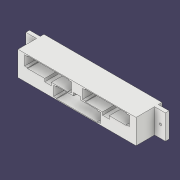
# Autodesk Inventor part: BP011
Saved by Autodesk Inventor 2017 SP1 (Build 210196100, 196)
## iProperties
Created: 2018-06-18
Part Number: BP011
Material: ABS Plastic
Document SubType Name: Modeling
Designer: Zach
Density: 1.06 g/cm^3
Appearance: CR White
Author: Zach
Autodesk Inventor part; units mm, degrees
ref_plane "YZ Plane" through (0, 0, 0) normal (1, 0, 0) x (0, 1, 0)
ref_plane "XZ Plane" through (0, 0, 0) normal (0, 1, 0) x (-1, 0, 0)
ref_plane "XY Plane" through (0, 0, 0) normal (0, 0, 1) x (1, 0, 0)
sketch "Sketch1" plane through (0, 0, 0) normal (0, 0, 1) x (1, 0, 0)
  line L0 (0, 0) -> (190, 0)
  line L1 (190, 0) -> (190, 35)
  line L2 (190, 35) -> (0, 35)
  line L3 (0, 35) -> (0, 0)
  circle A0 centre (7.5, 17.5) radius 1.5
  circle A1 centre (182.5, 17.5) radius 1.5
  point P0 (0, 17.5)
  dimension "d0" = 190
  dimension "d1" = 35
  dimension "d2" = 3
  dimension "d3" = 7.5
  dimension "d4" = 3
  dimension "d5" = 7.5
  constraints: 8 end point, 2 centre point, 2 horizontal alignment, 2 parallel, 1 horizontal, 1 midpoint, 1 perpendicular
  measures "d0" distance of L2.end L1.end
  measures "d1" distance of L1.end L0.end
  measures "d2" diameter of A0
  measures "d3" distance from line of L3 A0.centre
  measures "d4" diameter of A1
  measures "d5" distance from line of L1 A1.centre
extrude "Extrusion1" add sketch "Sketch1" along normal blind 5
sketch "Sketch2" plane through (0, 0, 0) normal (0, 0, -1) x (-1, 0, 0)
  line L0 (0, 0) -> (-190, 0) projected
  line L1 (-190, 35) -> (0, 35) projected
  line L2 (-15.5, 0) -> (-174.5, 0)
  line L3 (-174.5, 0) -> (-174.5, 35)
  line L4 (-174.5, 35) -> (-15.5, 35)
  line L5 (-15.5, 35) -> (-15.5, 0)
  point P0 (-95, 0)
  dimension "d8" = 159
  constraints: 8 end point, 2 midpoint, 2 parallel, 2 point on line, 1 horizontal, 1 perpendicular
  measures "d8" distance between parallel lines of L5 L3
extrude "Extrusion2" add sketch "Sketch2" along normal blind 5
sketch "Sketch3" plane through (0, 0, 5) normal (0, 0, 1) x (1, 0, 0)
  circle A0 centre (182.5, 17.5) radius 1.5 projected
  circle A1 centre (7.5, 17.5) radius 1.5 projected
  line L0 (0, 0) -> (190, 0) projected
  line L1 (190, 0) -> (190, 35) projected
  line L2 (190, 35) -> (0, 35) projected
  line L3 (0, 35) -> (0, 0) projected
  line L4 (1, 34) -> (189, 34)
  line L5 (189, 34) -> (189, 1)
  line L6 (189, 1) -> (1, 1)
  line L7 (1, 1) -> (1, 34)
  dimension "d11" = 1
  constraints: 8 end point, 3 other
  measures "d11" distance between parallel lines of L2 L4
extrude "Extrusion3" cut sketch "Sketch3" against normal through all contours L3 L2 L1 L0
sketch "Sketch4" plane through (0, 0, 5) normal (0, 0, 1) x (1, 0, 0)
  line L0 (41, 27) -> (71, 27)
  line L1 (71, 27) -> (71, 8)
  line L2 (71, 8) -> (41, 8)
  line L3 (41, 8) -> (41, 27)
  line L4 (86, 27) -> (116, 27)
  line L5 (116, 27) -> (116, 8)
  line L6 (116, 8) -> (86, 8)
  line L7 (86, 8) -> (86, 27)
  line L8 (131, 27) -> (149, 27)
  line L9 (149, 27) -> (149, 8)
  line L10 (149, 8) -> (131, 8)
  line L11 (131, 8) -> (131, 27)
  line L12 (41, 17.5) -> (149, 17.5) construction
  line L13 (189, 34) -> (1, 34) projected
  circle A0 centre (7.5, 17.5) radius 1.5 projected
  point P0 (0, 0)
  point P1 (95, 17.5)
  point P2 (95, 34)
  dimension "d14" = 30
  dimension "d15" = 19
  dimension "d16" = 30
  dimension "d17" = 19
  dimension "d18" = 18
  dimension "d19" = 19
  dimension "d20" = 15
  dimension "d21" = 15
  constraints: 26 end point, 6 parallel, 4 midpoint, 3 horizontal, 3 perpendicular, 2 point on line, 1 horizontal alignment, 1 vertical alignment
  measures "d14" distance of L1.end L2.end
  measures "d15" distance of L0.end L1.end
  measures "d16" distance of L5.end L6.end
  measures "d17" distance of L4.end L5.end
  measures "d18" distance of L9.end L10.end
  measures "d19" distance of L8.end L9.end
  measures "d20" distance between parallel lines of L1 L7
  measures "d21" distance between parallel lines of L11 L5
extrude "Extrusion4" cut sketch "Sketch4" against normal through all contours L0 L1 L2 L3 | L4 L5 L6 L7 | L8 L9 L10 L11
sketch "Sketch5" plane through (0, 0, 5) normal (0, 0, 1) x (1, 0, 0)
  line L0 (41, 27) -> (41, 8) projected
  line L1 (41, 8) -> (71, 8) projected
  line L2 (71, 8) -> (71, 27) projected
  line L3 (71, 27) -> (41, 27) projected
  line L4 (131, 27) -> (131, 8) projected
  line L5 (131, 8) -> (149, 8) projected
  line L6 (149, 8) -> (149, 27) projected
  line L7 (149, 27) -> (131, 27) projected
  line L8 (86, 27) -> (86, 8) projected
  line L9 (86, 8) -> (116, 8) projected
  line L10 (116, 8) -> (116, 27) projected
  line L11 (116, 27) -> (86, 27) projected
  line L12 (174.5, 1) -> (15.5, 1) projected
  line L13 (15.5, 1) -> (15.5, 34) projected
  line L14 (15.5, 34) -> (174.5, 34) projected
  line L15 (174.5, 34) -> (174.5, 1) projected
  point P0 (0, 0)
extrude "Extrusion5" add sketch "Sketch5" along normal blind 25
sketch "Sketch6" plane through (0, 0, -5) normal (0, 0, -1) x (-1, 0, 0)
  line L0 (-71, 27) -> (-41, 27) projected
  line L1 (-41, 27) -> (-41, 8) projected
  line L2 (-71, 8) -> (-71, 27) projected
  line L3 (-86, 27) -> (-86, 8) projected
  line L4 (-116, 27) -> (-86, 27) projected
  line L5 (-116, 8) -> (-116, 27) projected
  line L6 (-41, 25) -> (-36, 25)
  line L7 (-36, 25) -> (-36, 10)
  line L8 (-36, 10) -> (-41, 10)
  line L9 (-41, 10) -> (-41, 25)
  line L10 (-71, 25) -> (-76, 25)
  line L11 (-76, 25) -> (-76, 10)
  line L12 (-76, 10) -> (-71, 10)
  line L13 (-71, 10) -> (-71, 25)
  line L14 (-86, 25) -> (-81, 25)
  line L15 (-81, 25) -> (-81, 10)
  line L16 (-81, 10) -> (-86, 10)
  line L17 (-86, 10) -> (-86, 25)
  line L18 (-116, 25) -> (-121, 25)
  line L19 (-121, 25) -> (-121, 10)
  line L20 (-121, 10) -> (-116, 10)
  line L21 (-116, 10) -> (-116, 25)
  point P0 (0, 0)
  point P1 (-41, 17.5)
  dimension "d26" = 15
  dimension "d27" = 5
  dimension "d28" = 5
  dimension "d29" = 5
  dimension "d30" = 5
  constraints: 32 end point, 8 parallel, 6 horizontal alignment, 4 horizontal, 4 perpendicular, 4 point on line, 2 midpoint
  measures "d26" distance of L6.end L7.end
  measures "d27" distance of L6.start L6.end
  measures "d28" distance of L10.start L10.end
  measures "d29" distance of L14.start L14.end
  measures "d30" distance of L18.start L18.end
extrude "Extrusion6" cut sketch "Sketch6" against normal blind 22
sketch "Sketch10" plane through (0, 0, 30) normal (0, 0, 1) x (1, 0, 0)
  line L0 (86, 27) -> (116, 27) projected
  line L1 (116, 27) -> (116, 8) projected
  line L2 (116, 8) -> (86, 8) projected
  line L3 (86, 8) -> (86, 27) projected
  line L4 (41, 27) -> (71, 27) projected
  line L5 (71, 27) -> (71, 8) projected
  line L6 (71, 8) -> (41, 8) projected
  line L7 (41, 8) -> (41, 27) projected
  line L8 (131, 27) -> (149, 27) projected
  line L9 (149, 27) -> (149, 8) projected
  line L10 (149, 8) -> (131, 8) projected
  line L11 (131, 8) -> (131, 27) projected
  line L12 (15.5, 1) -> (174.5, 1) projected
  line L13 (174.5, 1) -> (174.5, 34) projected
  line L14 (174.5, 34) -> (15.5, 34) projected
  line L15 (15.5, 34) -> (15.5, 1) projected
  point P0 (0, 0)
extrude "Extrusion7" add sketch "Sketch10" against normal blind 35 contours L0 L1 L2 L3 | L4 L5 L6 L7 | L8 L9 L10 L11 | L15 L14 L13 L12
sketch "Sketch11" plane through (0, 0, 30) normal (0, 0, 1) x (1, 0, 0)
  line L0 (29.5, 32) -> (82.5, 32)
  line L1 (82.5, 32) -> (82.5, 19)
  line L2 (82.5, 19) -> (29.5, 19)
  line L3 (29.5, 19) -> (29.5, 32)
  line L4 (107.5, 32) -> (160.5, 32)
  line L5 (160.5, 32) -> (160.5, 19)
  line L6 (160.5, 19) -> (107.5, 19)
  line L7 (107.5, 19) -> (107.5, 32)
  line L8 (29.5, 32) -> (160.5, 32)
  line L9 (174.5, 34) -> (15.5, 34) projected
  line L10 (29.5, 32) -> (29.5, 3)
  line L11 (15.5, 34) -> (15.5, 1) projected
  line L12 (52.5, 19) -> (59.5, 19)
  line L13 (59.5, 19) -> (59.5, 15)
  line L14 (59.5, 15) -> (52.5, 15)
  line L15 (52.5, 15) -> (52.5, 19)
  line L16 (130.5, 19) -> (137.5, 19)
  line L17 (137.5, 19) -> (137.5, 15)
  line L18 (137.5, 15) -> (130.5, 15)
  line L19 (130.5, 15) -> (130.5, 19)
  line L20 (68.5, 3) -> (121.5, 3)
  line L21 (121.5, 3) -> (121.5, 16)
  line L22 (121.5, 16) -> (68.5, 16)
  line L23 (68.5, 16) -> (68.5, 3)
  line L24 (91.5, 16) -> (98.5, 16)
  line L25 (98.5, 16) -> (98.5, 20)
  line L26 (98.5, 20) -> (91.5, 20)
  line L27 (91.5, 20) -> (91.5, 16)
  point P0 (0, 0)
  point P1 (95, 32)
  point P2 (95, 34)
  point P3 (29.5, 17.5)
  point P4 (15.5, 17.5)
  point P5 (56, 19)
  point P6 (134, 19)
  point P7 (95, 16)
  point P8 (95, 20)
  dimension "d40" = 53
  dimension "d41" = 13
  dimension "d42" = 53
  dimension "d43" = 13
  dimension "d46" = 25
  dimension "d48" = 7
  dimension "d49" = 7
  dimension "d50" = 4
  dimension "d53" = 53
  dimension "d54" = 13
  dimension "d55" = 7
  dimension "d56" = 4
  dimension "d57" = 3
  dimension "d58" = 4
  constraints: 52 end point, 12 parallel, 11 midpoint, 6 horizontal, 6 perpendicular, 4 point on line, 3 horizontal alignment, 2 vertical alignment
  measures "d40" distance of L1.end L2.end
  measures "d41" distance of L2.end L0.start
  measures "d42" distance of L5.end L6.end
  measures "d43" distance of L6.end L4.start
  measures "d46" distance between parallel lines of L7 L1
  measures "d48" distance between parallel lines of L15 L13
  measures "d49" distance of L17.end L18.end
  measures "d50" distance of L16.end L17.end
  measures "d53" distance of L22.end L21.end
  measures "d54" distance of L21.end L20.end
  measures "d55" distance of L26.end L25.end
  measures "d56" distance of L25.end L24.end
  measures "d57" distance between parallel lines of L2 L22
  measures "d58" distance of L14.end L12.start
extrude "Extrusion8" cut sketch "Sketch11" against normal through all
sketch "Sketch13" plane through (0, 0, 30) normal (0, 0, 1) x (1, 0, 0)
  line L0 (98.5, 16) -> (121.5, 16) projected
  line L1 (121.5, 16) -> (121.5, 3) projected
  line L2 (121.5, 3) -> (68.5, 3) projected
  line L3 (68.5, 3) -> (68.5, 16) projected
  line L4 (68.5, 16) -> (91.5, 16) projected
  line L5 (91.5, 16) -> (91.5, 20) projected
  line L6 (91.5, 20) -> (98.5, 20) projected
  line L7 (98.5, 20) -> (98.5, 16) projected
  line L8 (52.5, 19) -> (29.5, 19) projected
  line L9 (29.5, 19) -> (29.5, 32) projected
  line L10 (29.5, 32) -> (82.5, 32) projected
  line L11 (82.5, 32) -> (82.5, 19) projected
  line L12 (82.5, 19) -> (59.5, 19) projected
  line L13 (59.5, 19) -> (59.5, 15) projected
  line L14 (59.5, 15) -> (52.5, 15) projected
  line L15 (52.5, 15) -> (52.5, 19) projected
  line L16 (130.5, 19) -> (107.5, 19) projected
  line L17 (107.5, 19) -> (107.5, 32) projected
  line L18 (107.5, 32) -> (160.5, 32) projected
  line L19 (160.5, 32) -> (160.5, 19) projected
  line L20 (160.5, 19) -> (137.5, 19) projected
  line L21 (137.5, 19) -> (137.5, 15) projected
  line L22 (137.5, 15) -> (130.5, 15) projected
  line L23 (130.5, 15) -> (130.5, 19) projected
  line L24 (15.5, 1) -> (174.5, 1) projected
  line L25 (174.5, 1) -> (174.5, 34) projected
  line L26 (174.5, 34) -> (15.5, 34) projected
  line L27 (15.5, 34) -> (15.5, 1) projected
  point P0 (0, 0)
extrude "Extrusion10" cut sketch "Sketch13" against normal blind 25
sketch "Sketch17" plane through (0, 0, 5) normal (0, 0, 1) x (1, 0, 0)
  circle A0 centre (7.5, 17.5) radius 1.5 projected
  line L0 (130.5, 19) -> (130.5, 15) projected
  line L1 (107.5, 19) -> (130.5, 19) projected
  line L2 (107.5, 32) -> (107.5, 19) projected
  line L3 (160.5, 32) -> (107.5, 32) projected
  line L4 (160.5, 19) -> (160.5, 32) projected
  line L5 (137.5, 19) -> (160.5, 19) projected
  line L6 (137.5, 15) -> (137.5, 19) projected
  line L7 (130.5, 15) -> (137.5, 15) projected
  line L8 (52.5, 19) -> (52.5, 15) projected
  line L9 (29.5, 19) -> (52.5, 19) projected
  line L10 (29.5, 32) -> (29.5, 19) projected
  line L11 (82.5, 32) -> (29.5, 32) projected
  line L12 (82.5, 19) -> (82.5, 32) projected
  line L13 (59.5, 19) -> (82.5, 19) projected
  line L14 (59.5, 15) -> (59.5, 19) projected
  line L15 (52.5, 15) -> (59.5, 15) projected
  line L16 (98.5, 16) -> (98.5, 20) projected
  line L17 (121.5, 16) -> (98.5, 16) projected
  line L18 (121.5, 3) -> (121.5, 16) projected
  line L19 (68.5, 3) -> (121.5, 3) projected
  line L20 (68.5, 16) -> (68.5, 3) projected
  line L21 (91.5, 16) -> (68.5, 16) projected
  line L22 (91.5, 20) -> (91.5, 16) projected
  line L23 (98.5, 20) -> (91.5, 20) projected
  circle A1 centre (182.5, 17.5) radius 1.5 projected
  line L24 (1, 1) -> (189, 1) projected
  line L25 (189, 1) -> (189, 34) projected
  line L26 (189, 34) -> (1, 34) projected
  line L27 (1, 34) -> (1, 1) projected
  line L28 (82.5, 32) -> (29.5, 32) projected
  line L29 (29.5, 32) -> (24.5, 32)
  line L30 (24.5, 32) -> (24.5, 19)
  line L31 (24.5, 19) -> (29.5, 19)
  line L32 (29.5, 19) -> (29.5, 32)
  line L33 (82.5, 32) -> (87.5, 32)
  line L34 (87.5, 32) -> (87.5, 19)
  line L35 (87.5, 19) -> (82.5, 19)
  line L36 (82.5, 19) -> (82.5, 32)
  line L37 (107.5, 32) -> (107.5, 19) projected
  line L38 (107.5, 32) -> (102.5, 32)
  line L39 (102.5, 32) -> (102.5, 19)
  line L40 (102.5, 19) -> (107.5, 19)
  line L41 (107.5, 19) -> (107.5, 32)
  line L42 (160.5, 32) -> (165.5, 32)
  line L43 (165.5, 32) -> (165.5, 19)
  line L44 (165.5, 19) -> (160.5, 19)
  line L45 (160.5, 19) -> (160.5, 32)
  line L46 (121.5, 16) -> (98.5, 16) projected
  line L47 (121.5, 16) -> (126.5, 16)
  line L48 (126.5, 16) -> (126.5, 3)
  line L49 (126.5, 3) -> (121.5, 3)
  line L50 (121.5, 3) -> (121.5, 16)
  line L51 (68.5, 16) -> (63.5, 16)
  line L52 (63.5, 16) -> (63.5, 3)
  line L53 (63.5, 3) -> (68.5, 3)
  line L54 (68.5, 3) -> (68.5, 16)
  line L55 (15.5, 34) -> (15.5, 1) projected
  line L56 (174.5, 1) -> (174.5, 34) projected
  point P0 (0, 0)
  point P1 (95, 3)
  dimension "d84" = 5
  dimension "d85" = 5
  dimension "d86" = 5
  dimension "d87" = 5
  dimension "d88" = 5
  dimension "d89" = 5
  constraints: 48 end point, 12 parallel, 6 horizontal, 6 perpendicular, 4 point on line, 2 horizontal alignment, 1 midpoint
  measures "d84" distance of L31.end L30.end
  measures "d85" distance of L34.end L35.end
  measures "d86" distance of L40.end L39.end
  measures "d87" distance of L43.end L44.end
  measures "d88" distance of L48.end L49.end
  measures "d89" distance of L53.end L52.end
extrude "Extrusion15" add sketch "Sketch17" along normal blind 25 contours L17 L18 L19 L20 L21 L22 L23 L16 | L55 L26 L56 L24
sketch "Sketch19" plane through (0, 0, 5) normal (0, 0, 1) x (1, 0, 0)
  line L0 (121.5, 16) -> (98.5, 16) projected
  line L1 (98.5, 16) -> (98.5, 20) projected
  line L2 (98.5, 20) -> (91.5, 20) projected
  line L3 (91.5, 20) -> (91.5, 16) projected
  line L4 (91.5, 16) -> (68.5, 16) projected
  line L5 (68.5, 16) -> (68.5, 3) projected
  line L6 (68.5, 3) -> (121.5, 3) construction
  line L7 (121.5, 3) -> (121.5, 16) projected
  line L8 (29.5, 19) -> (52.5, 19) projected
  line L9 (52.5, 19) -> (52.5, 15) projected
  line L10 (52.5, 15) -> (59.5, 15) projected
  line L11 (59.5, 15) -> (59.5, 19) projected
  line L12 (59.5, 19) -> (82.5, 19) projected
  line L13 (82.5, 19) -> (82.5, 32) projected
  line L14 (82.5, 32) -> (29.5, 32) construction
  line L15 (29.5, 32) -> (29.5, 19) projected
  line L16 (107.5, 19) -> (130.5, 19) projected
  line L17 (130.5, 19) -> (130.5, 15) projected
  line L18 (130.5, 15) -> (137.5, 15) projected
  line L19 (137.5, 15) -> (137.5, 19) projected
  line L20 (137.5, 19) -> (160.5, 19) projected
  line L21 (160.5, 19) -> (160.5, 32) projected
  line L22 (160.5, 32) -> (107.5, 32) construction
  line L23 (107.5, 32) -> (107.5, 19) projected
  line L24 (174.5, 1) -> (15.5, 1) projected
  line L25 (15.5, 1) -> (15.5, 34) projected
  line L26 (15.5, 34) -> (174.5, 34) construction
  line L27 (174.5, 34) -> (174.5, 1) projected
  line L28 (83.5, 33) -> (83.5, 18)
  line L29 (83.5, 18) -> (60.5, 18)
  line L30 (60.5, 18) -> (60.5, 14)
  line L31 (60.5, 14) -> (51.5, 14)
  line L32 (51.5, 14) -> (51.5, 18)
  line L33 (51.5, 18) -> (28.5, 18)
  line L34 (28.5, 18) -> (28.5, 33)
  line L35 (28.5, 33) -> (83.5, 33)
  line L36 (67.5, 17) -> (90.5, 17)
  line L37 (90.5, 17) -> (90.5, 21)
  line L38 (90.5, 21) -> (99.5, 21)
  line L39 (99.5, 21) -> (99.5, 17)
  line L40 (99.5, 17) -> (122.5, 17)
  line L41 (122.5, 17) -> (122.5, 2)
  line L42 (122.5, 2) -> (67.5, 2)
  line L43 (67.5, 2) -> (67.5, 17)
  line L44 (106.5, 18) -> (129.5, 18)
  line L45 (129.5, 18) -> (129.5, 14)
  line L46 (129.5, 14) -> (138.5, 14)
  line L47 (138.5, 14) -> (138.5, 18)
  line L48 (138.5, 18) -> (161.5, 18)
  line L49 (161.5, 18) -> (161.5, 33)
  line L50 (161.5, 33) -> (106.5, 33)
  line L51 (106.5, 33) -> (106.5, 18)
  point P0 (0, 0)
  dimension "d93" = 1
  dimension "d94" = 1
  dimension "d95" = 1
  constraints: 48 end point, 21 other
  measures "d93" distance between parallel lines of L13 L28
  measures "d94" distance between parallel lines of L4 L36
  measures "d95" distance between parallel lines of L23 L51
extrude "Extrusion16" cut sketch "Sketch19" along normal through all
sketch "Sketch20" plane through (0, 0, 5) normal (0, 0, 1) x (1, 0, 0)
  line L0 (29.5, 32) -> (29.5, 19) projected
  line L1 (82.5, 32) -> (29.5, 32) projected
  line L2 (82.5, 19) -> (82.5, 32) construction
  line L3 (59.5, 19) -> (82.5, 19) projected
  line L4 (59.5, 15) -> (59.5, 19) projected
  line L5 (52.5, 15) -> (59.5, 15) projected
  line L6 (52.5, 19) -> (52.5, 15) projected
  line L7 (29.5, 19) -> (52.5, 19) projected
  line L8 (28.5, 18) -> (28.5, 19) projected
  line L9 (51.5, 18) -> (28.5, 18) projected
  line L10 (51.5, 14) -> (51.5, 18) projected
  line L11 (60.5, 14) -> (51.5, 14) construction
  line L12 (60.5, 18) -> (60.5, 14) projected
  line L13 (83.5, 18) -> (60.5, 18) projected
  line L14 (83.5, 19) -> (83.5, 18) projected
  line L15 (83.5, 19) -> (87.5, 19) projected
  line L16 (87.5, 19) -> (87.5, 32) projected
  line L17 (87.5, 32) -> (83.5, 32) projected
  line L18 (83.5, 33) -> (83.5, 32) projected
  line L19 (28.5, 33) -> (83.5, 33) projected
  line L20 (28.5, 32) -> (28.5, 33) projected
  line L21 (28.5, 32) -> (24.5, 32) projected
  line L22 (24.5, 32) -> (24.5, 19) projected
  line L23 (24.5, 19) -> (28.5, 19) projected
  line L24 (121.5, 3) -> (121.5, 16) construction
  line L25 (68.5, 3) -> (121.5, 3) projected
  line L26 (68.5, 16) -> (68.5, 3) projected
  line L27 (91.5, 16) -> (68.5, 16) projected
  line L28 (91.5, 20) -> (91.5, 16) projected
  line L29 (98.5, 20) -> (91.5, 20) projected
  line L30 (98.5, 16) -> (98.5, 20) projected
  line L31 (121.5, 16) -> (98.5, 16) projected
  line L32 (122.5, 17) -> (122.5, 16) projected
  line L33 (99.5, 17) -> (122.5, 17) projected
  line L34 (99.5, 21) -> (99.5, 17) projected
  line L35 (90.5, 21) -> (99.5, 21) construction
  line L36 (90.5, 17) -> (90.5, 21) projected
  line L37 (67.5, 17) -> (90.5, 17) projected
  line L38 (67.5, 16) -> (67.5, 17) projected
  line L39 (67.5, 16) -> (63.5, 16) projected
  line L40 (63.5, 16) -> (63.5, 3) projected
  line L41 (63.5, 3) -> (67.5, 3) projected
  line L42 (67.5, 2) -> (67.5, 3) projected
  line L43 (122.5, 2) -> (67.5, 2) projected
  line L44 (122.5, 3) -> (122.5, 2) projected
  line L45 (122.5, 3) -> (126.5, 3) projected
  line L46 (126.5, 3) -> (126.5, 16) projected
  line L47 (126.5, 16) -> (122.5, 16) projected
  line L48 (107.5, 32) -> (107.5, 19) construction
  line L49 (160.5, 32) -> (107.5, 32) projected
  line L50 (160.5, 19) -> (160.5, 32) projected
  line L51 (137.5, 19) -> (160.5, 19) projected
  line L52 (137.5, 15) -> (137.5, 19) projected
  line L53 (130.5, 15) -> (137.5, 15) projected
  line L54 (130.5, 19) -> (130.5, 15) projected
  line L55 (107.5, 19) -> (130.5, 19) projected
  line L56 (106.5, 19) -> (106.5, 18) projected
  line L57 (106.5, 18) -> (129.5, 18) construction
  line L58 (129.5, 18) -> (129.5, 14) projected
  line L59 (129.5, 14) -> (138.5, 14) projected
  line L60 (138.5, 14) -> (138.5, 18) projected
  line L61 (138.5, 18) -> (161.5, 18) projected
  line L62 (161.5, 18) -> (161.5, 19) projected
  line L63 (161.5, 19) -> (165.5, 19) projected
  line L64 (165.5, 19) -> (165.5, 32) projected
  line L65 (165.5, 32) -> (161.5, 32) projected
  line L66 (161.5, 32) -> (161.5, 33) projected
  line L67 (161.5, 33) -> (106.5, 33) projected
  line L68 (106.5, 33) -> (106.5, 32) projected
  line L69 (106.5, 32) -> (102.5, 32) projected
  line L70 (102.5, 32) -> (102.5, 19) projected
  line L71 (102.5, 19) -> (106.5, 19) projected
  line L72 (68.5, 16) -> (68.5, 3) projected
  line L73 (121.5, 3) -> (68.5, 3)
  line L74 (68.5, 3) -> (68.5, 4)
  line L75 (68.5, 4) -> (121.5, 4)
  line L76 (121.5, 4) -> (121.5, 3)
  line L77 (68.5, 16) -> (121.5, 16)
  line L78 (121.5, 16) -> (121.5, 15)
  line L79 (121.5, 15) -> (68.5, 15)
  line L80 (68.5, 15) -> (68.5, 16)
  line L81 (29.5, 32) -> (29.5, 19) projected
  line L82 (82.5, 19) -> (29.5, 19)
  line L83 (29.5, 19) -> (29.5, 20)
  line L84 (29.5, 20) -> (82.5, 20)
  line L85 (82.5, 20) -> (82.5, 19)
  line L86 (82.5, 19) -> (82.5, 32) projected
  line L87 (29.5, 32) -> (82.5, 32)
  line L88 (82.5, 32) -> (82.5, 31)
  line L89 (82.5, 31) -> (29.5, 31)
  line L90 (29.5, 31) -> (29.5, 32)
  line L91 (137.5, 19) -> (160.5, 19) projected
  line L92 (107.5, 32) -> (107.5, 19) projected
  line L93 (160.5, 19) -> (107.5, 19)
  line L94 (107.5, 19) -> (107.5, 20)
  line L95 (107.5, 20) -> (160.5, 20)
  line L96 (160.5, 20) -> (160.5, 19)
  line L97 (107.5, 32) -> (160.5, 32)
  line L98 (160.5, 32) -> (160.5, 31)
  line L99 (160.5, 31) -> (107.5, 31)
  line L100 (107.5, 31) -> (107.5, 32)
  line L101 (121.5, 16) -> (98.5, 16) projected
  line L102 (91.5, 16) -> (68.5, 16) projected
  line L103 (91.5, 16) -> (91.5, 15)
  line L104 (137.5, 15) -> (137.5, 19) projected
  line L105 (137.5, 19) -> (137.5, 20)
  line L106 (130.5, 19) -> (130.5, 15) projected
  line L107 (130.5, 19) -> (130.5, 20)
  line L108 (59.5, 19) -> (59.5, 20)
  line L109 (29.5, 19) -> (52.5, 19) projected
  line L110 (52.5, 19) -> (52.5, 20)
  line L111 (98.5, 15) -> (98.5, 16)
  point P0 (0, 0)
  dimension "d98" = 1
  dimension "d99" = 1
  dimension "d100" = 1
  dimension "d101" = 1
  dimension "d102" = 1
  dimension "d103" = 1
  constraints: 60 end point, 13 point on line, 12 parallel, 11 perpendicular, 6 horizontal, 1 collinear, 1 vertical alignment
  measures "d98" distance between parallel lines of L25 L75
  measures "d99" distance between parallel lines of L27 L79
  measures "d100" distance between parallel lines of L82 L84
  measures "d101" distance between parallel lines of L1 L89
  measures "d102" distance between parallel lines of L93 L95
  measures "d103" distance between parallel lines of L97 L99
extrude "Extrusion17" add sketch "Sketch20" against normal blind 3 contours L1 L86 L89 L0 | L84 L110 L7 L0 | L85 L3 L108 L84 | L26 L75 L76 L25 | L27 L103 L79 L26 | L31 L78 L79 L111 | L50 L99 L92 L49 | L50 L51 L105 L95 | L95 L107 L55 L92
body "Solid1"
